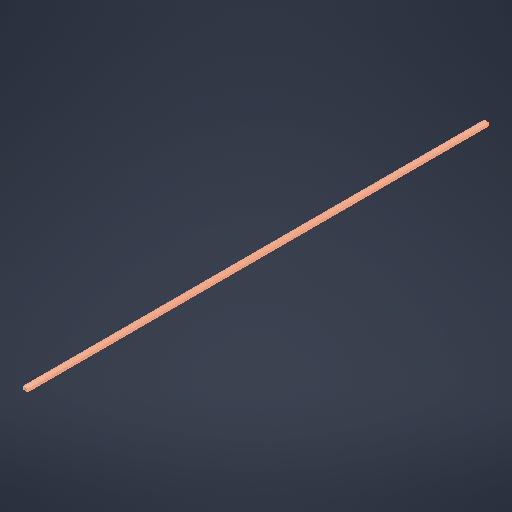
# Autodesk Inventor part: WOOD_STOCK_TREBUCHET
Saved by Autodesk Inventor 2026.2 (Build 302298010, 298A)
## iProperties
Created: 2026-02-12
Part Number: WOOD_STOCK_TREBUCHET
Material: Wood (Oak)
Document SubType Name: Modeling
Designer: 4aida
Density: 0.76 g/cm^3
Appearance: White Oak - Natural Medium Gloss
Author: 4aida
Autodesk Inventor part; units mm, degrees
ref_plane "YZ Plane" through (0, 0, 0) normal (1, 0, 0) x (0, 1, 0)
ref_plane "XZ Plane" through (0, 0, 0) normal (0, 1, 0) x (-1, 0, 0)
ref_plane "XY Plane" through (0, 0, 0) normal (0, 0, 1) x (1, 0, 0)
sketch "Sketch1" plane through (0, 0, 0) normal (0, 1, 0) x (-1, 0, 0)
  line L0 (-9.525, -914.4) -> (9.525, -914.4)
  line L1 (9.525, -914.4) -> (9.525, 914.4)
  line L2 (9.525, 914.4) -> (-9.525, 914.4)
  line L3 (-9.525, 914.4) -> (-9.525, -914.4)
  line L4 (-9.525, -914.4) -> (9.525, 914.4) construction
  line L5 (9.525, -914.4) -> (-9.525, 914.4) construction
  point P0 (0, 0)
  dimension "d0" = 19.05
  dimension "d1" = 1828.8
  constraints: 12 end point, 2 midpoint, 2 parallel, 1 horizontal, 1 perpendicular
  measures "d0" distance of L2.end L1.end
  measures "d1" distance of L1.end L0.end
extrude "Extrusion1" add sketch "Sketch1" along normal mid plane 9.525
body "Solid1"
